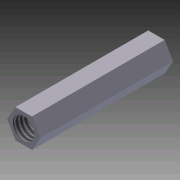
# Autodesk Inventor part: Traction Wheel Brace 1764
Saved by Autodesk Inventor 2011 (Build 150239000, 239)
## iProperties
Created: 2009-01-17
Part Number: Traction Wheel Brace 1764
Document SubType Name: Modeling
Designer: pmulligan
Density: 1 g/cm^3
Mass: 0.671375 g
Surface Area: 16.9086 cm^2
Volume: 0.671375 cm^3
Author: pmulligan
Autodesk Inventor part; units mm, degrees
ref_plane "YZ Plane" through (0, 0, 0) normal (1, 0, 0) x (0, 1, 0)
ref_plane "XZ Plane" through (0, 0, 0) normal (0, 1, 0) x (-1, 0, 0)
ref_plane "XY Plane" through (0, 0, 0) normal (0, 0, 1) x (1, 0, 0)
sketch "Sketch1" plane through (0, 0, 0) normal (0, 0, 1) x (1, 0, 0)
  line L0 (-23.1568, 23.3878) -> (-24.7235, 20.6262)
  line L1 (-24.7235, 20.6262) -> (-27.8985, 20.6021)
  line L2 (-27.8985, 20.6021) -> (-29.5068, 23.3397)
  line L3 (-29.5068, 23.3397) -> (-27.9402, 26.1014)
  line L4 (-27.9402, 26.1014) -> (-24.7652, 26.1254)
  line L5 (-24.7652, 26.1254) -> (-23.1568, 23.3878)
  circle A0 centre (-26.3318, 23.3638) radius 2.0574
  dimension "d0" = 6.35
  dimension "d1" = 4.1148
  constraints: 12 end point, 1 centre point, 1 coincident, 13 other
  measures "d0" horizontal distance of L0.start L2.end
  measures "d1" diameter of A0
extrude "Extrusion1" add sketch "Sketch1" along normal blind 25.4
thread "Thread1" size "8-32 UNC" class "2B" standard "ANSI Unified Screw Threads" full length
body "Solid1"
